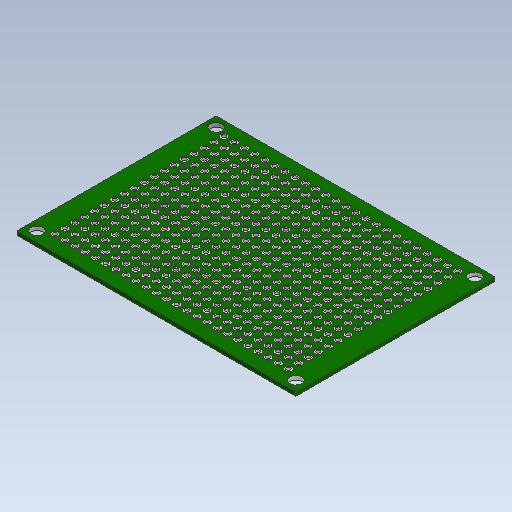
# Autodesk Inventor part: Lochrasterplatine50x70
Saved by Autodesk Inventor 2021 (Build 250183000, 183)
## iProperties
Created: 2020-12-16
Part Number: Lochrasterplatine50x70
Material: Generisch
Document SubType Name: Modeling
Designer: laure
Density: 1 g/cm^3
Appearance: Vorgabe
Author: laure
Autodesk Inventor part; units mm, degrees
(part 1 of 2)
ref_plane "YZ Plane" through (0, 0, 0) normal (1, 0, 0) x (0, 1, 0)
ref_plane "XZ Plane" through (0, 0, 0) normal (0, 1, 0) x (-1, 0, 0)
ref_plane "XY Plane" through (0, 0, 0) normal (0, 0, 1) x (1, 0, 0)
sketch "Skizze1" plane through (0, 0, 0) normal (0, 1, 0) x (-1, 0, 0)
  line L0 (-35, -25) -> (35, -25)
  line L1 (35, -25) -> (35, 25)
  line L2 (35, 25) -> (-35, 25)
  line L3 (-35, 25) -> (-35, -25)
  line L4 (0, -35) -> (0, 35) projected
  line L5 (49, 0) -> (-49, 0) projected
  point P0 (0, 0)
  dimension "d0" = 70
  dimension "d1" = 50
  constraints: 8 end point, 2 parallel, 1 horizontal, 1 perpendicular, 2 other
  measures "d0" distance of L1.end L2.end
  measures "d1" distance of L0.end L1.end
extrude "Extrusion1" add sketch "Skizze1" along normal mid plane 1
sketch "Skizze2" plane through (0, 0.5, 0) normal (0, 1, 0) x (1, 0, 0)
  circle A0 centre (-29.5, 21.5) radius 0.5
  line L0 (-35, 25) -> (-35, -25) projected
  line L1 (35, 25) -> (-35, 25) projected
  circle A1 centre (-26.95, 21.5) radius 0.5
  circle A2 centre (-24.4, 21.5) radius 0.5
  circle A3 centre (-21.85, 21.5) radius 0.5
  circle A4 centre (-19.3, 21.5) radius 0.5
  circle A5 centre (-16.75, 21.5) radius 0.5
  circle A6 centre (-14.2, 21.5) radius 0.5
  circle A7 centre (-11.65, 21.5) radius 0.5
  circle A8 centre (-9.1, 21.5) radius 0.5
  circle A9 centre (-6.55, 21.5) radius 0.5
  circle A10 centre (-4, 21.5) radius 0.5
  circle A11 centre (-1.45, 21.5) radius 0.5
  circle A12 centre (1.1, 21.5) radius 0.5
  circle A13 centre (3.65, 21.5) radius 0.5
  circle A14 centre (6.2, 21.5) radius 0.5
  circle A15 centre (8.75, 21.5) radius 0.5
  circle A16 centre (11.3, 21.5) radius 0.5
  circle A17 centre (13.85, 21.5) radius 0.5
  circle A18 centre (16.4, 21.5) radius 0.5
  circle A19 centre (18.95, 21.5) radius 0.5
  circle A20 centre (21.5, 21.5) radius 0.5
  circle A21 centre (24.05, 21.5) radius 0.5
  circle A22 centre (26.6, 21.5) radius 0.5
  circle A23 centre (29.15, 21.5) radius 0.5
  circle A24 centre (-29.5, 19) radius 0.5
  circle A25 centre (-26.95, 19) radius 0.5
  circle A26 centre (-24.4, 19) radius 0.5
  circle A27 centre (-21.85, 19) radius 0.5
  circle A28 centre (-19.3, 19) radius 0.5
  circle A29 centre (-16.75, 19) radius 0.5
  circle A30 centre (-14.2, 19) radius 0.5
  circle A31 centre (-11.65, 19) radius 0.5
  circle A32 centre (-9.1, 19) radius 0.5
  circle A33 centre (-6.55, 19) radius 0.5
  circle A34 centre (-4, 19) radius 0.5
  circle A35 centre (-1.45, 19) radius 0.5
  circle A36 centre (1.1, 19) radius 0.5
  circle A37 centre (3.65, 19) radius 0.5
  circle A38 centre (6.2, 19) radius 0.5
  circle A39 centre (8.75, 19) radius 0.5
  circle A40 centre (11.3, 19) radius 0.5
  circle A41 centre (13.85, 19) radius 0.5
  circle A42 centre (16.4, 19) radius 0.5
  circle A43 centre (18.95, 19) radius 0.5
  circle A44 centre (21.5, 19) radius 0.5
  circle A45 centre (24.05, 19) radius 0.5
  circle A46 centre (26.6, 19) radius 0.5
  circle A47 centre (29.15, 19) radius 0.5
  circle A48 centre (-29.5, 16.5) radius 0.5
  circle A49 centre (-26.95, 16.5) radius 0.5
  circle A50 centre (-24.4, 16.5) radius 0.5
  circle A51 centre (-21.85, 16.5) radius 0.5
  circle A52 centre (-19.3, 16.5) radius 0.5
  circle A53 centre (-16.75, 16.5) radius 0.5
  circle A54 centre (-14.2, 16.5) radius 0.5
  circle A55 centre (-11.65, 16.5) radius 0.5
  circle A56 centre (-9.1, 16.5) radius 0.5
  circle A57 centre (-6.55, 16.5) radius 0.5
  circle A58 centre (-4, 16.5) radius 0.5
  circle A59 centre (-1.45, 16.5) radius 0.5
  circle A60 centre (1.1, 16.5) radius 0.5
  circle A61 centre (3.65, 16.5) radius 0.5
  circle A62 centre (6.2, 16.5) radius 0.5
  circle A63 centre (8.75, 16.5) radius 0.5
  circle A64 centre (11.3, 16.5) radius 0.5
  circle A65 centre (13.85, 16.5) radius 0.5
  circle A66 centre (16.4, 16.5) radius 0.5
  circle A67 centre (18.95, 16.5) radius 0.5
  circle A68 centre (21.5, 16.5) radius 0.5
  circle A69 centre (24.05, 16.5) radius 0.5
  circle A70 centre (26.6, 16.5) radius 0.5
  circle A71 centre (29.15, 16.5) radius 0.5
  circle A72 centre (-29.5, 14) radius 0.5
  circle A73 centre (-26.95, 14) radius 0.5
  circle A74 centre (-24.4, 14) radius 0.5
  circle A75 centre (-21.85, 14) radius 0.5
  circle A76 centre (-19.3, 14) radius 0.5
  circle A77 centre (-16.75, 14) radius 0.5
  circle A78 centre (-14.2, 14) radius 0.5
  circle A79 centre (-11.65, 14) radius 0.5
  circle A80 centre (-9.1, 14) radius 0.5
  circle A81 centre (-6.55, 14) radius 0.5
  circle A82 centre (-4, 14) radius 0.5
  circle A83 centre (-1.45, 14) radius 0.5
  circle A84 centre (1.1, 14) radius 0.5
  circle A85 centre (3.65, 14) radius 0.5
  circle A86 centre (6.2, 14) radius 0.5
  circle A87 centre (8.75, 14) radius 0.5
  circle A88 centre (11.3, 14) radius 0.5
  circle A89 centre (13.85, 14) radius 0.5
  circle A90 centre (16.4, 14) radius 0.5
  circle A91 centre (18.95, 14) radius 0.5
  circle A92 centre (21.5, 14) radius 0.5
  circle A93 centre (24.05, 14) radius 0.5
  circle A94 centre (26.6, 14) radius 0.5
  circle A95 centre (29.15, 14) radius 0.5
  circle A96 centre (-29.5, 11.5) radius 0.5
  circle A97 centre (-26.95, 11.5) radius 0.5
  circle A98 centre (-24.4, 11.5) radius 0.5
  circle A99 centre (-21.85, 11.5) radius 0.5
  circle A100 centre (-19.3, 11.5) radius 0.5
  circle A101 centre (-16.75, 11.5) radius 0.5
  circle A102 centre (-14.2, 11.5) radius 0.5
  circle A103 centre (-11.65, 11.5) radius 0.5
  circle A104 centre (-9.1, 11.5) radius 0.5
  circle A105 centre (-6.55, 11.5) radius 0.5
  circle A106 centre (-4, 11.5) radius 0.5
  circle A107 centre (-1.45, 11.5) radius 0.5
  circle A108 centre (1.1, 11.5) radius 0.5
  circle A109 centre (3.65, 11.5) radius 0.5
  circle A110 centre (6.2, 11.5) radius 0.5
  circle A111 centre (8.75, 11.5) radius 0.5
  circle A112 centre (11.3, 11.5) radius 0.5
  circle A113 centre (13.85, 11.5) radius 0.5
  circle A114 centre (16.4, 11.5) radius 0.5
  circle A115 centre (18.95, 11.5) radius 0.5
  circle A116 centre (21.5, 11.5) radius 0.5
  circle A117 centre (24.05, 11.5) radius 0.5
  circle A118 centre (26.6, 11.5) radius 0.5
  circle A119 centre (29.15, 11.5) radius 0.5
  circle A120 centre (-29.5, 9) radius 0.5
  circle A121 centre (-26.95, 9) radius 0.5
  circle A122 centre (-24.4, 9) radius 0.5
  circle A123 centre (-21.85, 9) radius 0.5
  circle A124 centre (-19.3, 9) radius 0.5
  circle A125 centre (-16.75, 9) radius 0.5
  circle A126 centre (-14.2, 9) radius 0.5
  circle A127 centre (-11.65, 9) radius 0.5
  circle A128 centre (-9.1, 9) radius 0.5
  circle A129 centre (-6.55, 9) radius 0.5
  circle A130 centre (-4, 9) radius 0.5
  circle A131 centre (-1.45, 9) radius 0.5
  circle A132 centre (1.1, 9) radius 0.5
  circle A133 centre (3.65, 9) radius 0.5
  circle A134 centre (6.2, 9) radius 0.5
  circle A135 centre (8.75, 9) radius 0.5
  circle A136 centre (11.3, 9) radius 0.5
  circle A137 centre (13.85, 9) radius 0.5
  circle A138 centre (16.4, 9) radius 0.5
  circle A139 centre (18.95, 9) radius 0.5
  circle A140 centre (21.5, 9) radius 0.5
  circle A141 centre (24.05, 9) radius 0.5
  circle A142 centre (26.6, 9) radius 0.5
  circle A143 centre (29.15, 9) radius 0.5
  circle A144 centre (-29.5, 6.5) radius 0.5
  circle A145 centre (-26.95, 6.5) radius 0.5
  circle A146 centre (-24.4, 6.5) radius 0.5
  circle A147 centre (-21.85, 6.5) radius 0.5
  circle A148 centre (-19.3, 6.5) radius 0.5
  circle A149 centre (-16.75, 6.5) radius 0.5
  circle A150 centre (-14.2, 6.5) radius 0.5
  circle A151 centre (-11.65, 6.5) radius 0.5
  circle A152 centre (-9.1, 6.5) radius 0.5
  circle A153 centre (-6.55, 6.5) radius 0.5
  circle A154 centre (-4, 6.5) radius 0.5
  circle A155 centre (-1.45, 6.5) radius 0.5
  circle A156 centre (1.1, 6.5) radius 0.5
  circle A157 centre (3.65, 6.5) radius 0.5
  circle A158 centre (6.2, 6.5) radius 0.5
  circle A159 centre (8.75, 6.5) radius 0.5
  circle A160 centre (11.3, 6.5) radius 0.5
  circle A161 centre (13.85, 6.5) radius 0.5
  circle A162 centre (16.4, 6.5) radius 0.5
  circle A163 centre (18.95, 6.5) radius 0.5
  circle A164 centre (21.5, 6.5) radius 0.5
  circle A165 centre (24.05, 6.5) radius 0.5
  circle A166 centre (26.6, 6.5) radius 0.5
  circle A167 centre (29.15, 6.5) radius 0.5
  circle A168 centre (-29.5, 4) radius 0.5
  circle A169 centre (-26.95, 4) radius 0.5
  circle A170 centre (-24.4, 4) radius 0.5
  circle A171 centre (-21.85, 4) radius 0.5
  circle A172 centre (-19.3, 4) radius 0.5
  circle A173 centre (-16.75, 4) radius 0.5
  circle A174 centre (-14.2, 4) radius 0.5
  circle A175 centre (-11.65, 4) radius 0.5
  circle A176 centre (-9.1, 4) radius 0.5
  circle A177 centre (-6.55, 4) radius 0.5
  circle A178 centre (-4, 4) radius 0.5
  circle A179 centre (-1.45, 4) radius 0.5
  circle A180 centre (1.1, 4) radius 0.5
  circle A181 centre (3.65, 4) radius 0.5
  circle A182 centre (6.2, 4) radius 0.5
  circle A183 centre (8.75, 4) radius 0.5
  circle A184 centre (11.3, 4) radius 0.5
  circle A185 centre (13.85, 4) radius 0.5
  circle A186 centre (16.4, 4) radius 0.5
  circle A187 centre (18.95, 4) radius 0.5
  circle A188 centre (21.5, 4) radius 0.5
  circle A189 centre (24.05, 4) radius 0.5
  circle A190 centre (26.6, 4) radius 0.5
  circle A191 centre (29.15, 4) radius 0.5
  circle A192 centre (-29.5, 1.5) radius 0.5
  circle A193 centre (-26.95, 1.5) radius 0.5
  circle A194 centre (-24.4, 1.5) radius 0.5
  circle A195 centre (-21.85, 1.5) radius 0.5
  circle A196 centre (-19.3, 1.5) radius 0.5
  circle A197 centre (-16.75, 1.5) radius 0.5
  circle A198 centre (-14.2, 1.5) radius 0.5
  circle A199 centre (-11.65, 1.5) radius 0.5
  circle A200 centre (-9.1, 1.5) radius 0.5
  circle A201 centre (-6.55, 1.5) radius 0.5
  circle A202 centre (-4, 1.5) radius 0.5
  circle A203 centre (-1.45, 1.5) radius 0.5
  circle A204 centre (1.1, 1.5) radius 0.5
  circle A205 centre (3.65, 1.5) radius 0.5
  circle A206 centre (6.2, 1.5) radius 0.5
  circle A207 centre (8.75, 1.5) radius 0.5
  circle A208 centre (11.3, 1.5) radius 0.5
  circle A209 centre (13.85, 1.5) radius 0.5
  circle A210 centre (16.4, 1.5) radius 0.5
  circle A211 centre (18.95, 1.5) radius 0.5
  circle A212 centre (21.5, 1.5) radius 0.5
  circle A213 centre (24.05, 1.5) radius 0.5
  circle A214 centre (26.6, 1.5) radius 0.5
  circle A215 centre (29.15, 1.5) radius 0.5
  circle A216 centre (-29.5, -1) radius 0.5
  circle A217 centre (-26.95, -1) radius 0.5
  circle A218 centre (-24.4, -1) radius 0.5
  circle A219 centre (-21.85, -1) radius 0.5
  circle A220 centre (-19.3, -1) radius 0.5
  circle A221 centre (-16.75, -1) radius 0.5
  circle A222 centre (-14.2, -1) radius 0.5
  circle A223 centre (-11.65, -1) radius 0.5
  circle A224 centre (-9.1, -1) radius 0.5
  circle A225 centre (-6.55, -1) radius 0.5
  circle A226 centre (-4, -1) radius 0.5
  circle A227 centre (-1.45, -1) radius 0.5
  circle A228 centre (1.1, -1) radius 0.5
  circle A229 centre (3.65, -1) radius 0.5
  circle A230 centre (6.2, -1) radius 0.5
  circle A231 centre (8.75, -1) radius 0.5
  circle A232 centre (11.3, -1) radius 0.5
  circle A233 centre (13.85, -1) radius 0.5
  circle A234 centre (16.4, -1) radius 0.5
  circle A235 centre (18.95, -1) radius 0.5
  circle A236 centre (21.5, -1) radius 0.5
  circle A237 centre (24.05, -1) radius 0.5
  circle A238 centre (26.6, -1) radius 0.5
  circle A239 centre (29.15, -1) radius 0.5
  circle A240 centre (-29.5, -3.5) radius 0.5
  circle A241 centre (-26.95, -3.5) radius 0.5
  circle A242 centre (-24.4, -3.5) radius 0.5
  circle A243 centre (-21.85, -3.5) radius 0.5
  circle A244 centre (-19.3, -3.5) radius 0.5
  circle A245 centre (-16.75, -3.5) radius 0.5
  circle A246 centre (-14.2, -3.5) radius 0.5
  circle A247 centre (-11.65, -3.5) radius 0.5
  circle A248 centre (-9.1, -3.5) radius 0.5
  circle A249 centre (-6.55, -3.5) radius 0.5
  circle A250 centre (-4, -3.5) radius 0.5
  circle A251 centre (-1.45, -3.5) radius 0.5
  circle A252 centre (1.1, -3.5) radius 0.5
  circle A253 centre (3.65, -3.5) radius 0.5
  circle A254 centre (6.2, -3.5) radius 0.5
  circle A255 centre (8.75, -3.5) radius 0.5
  circle A256 centre (11.3, -3.5) radius 0.5
  circle A257 centre (13.85, -3.5) radius 0.5
  circle A258 centre (16.4, -3.5) radius 0.5
  circle A259 centre (18.95, -3.5) radius 0.5
  circle A260 centre (21.5, -3.5) radius 0.5
  circle A261 centre (24.05, -3.5) radius 0.5
  circle A262 centre (26.6, -3.5) radius 0.5
  circle A263 centre (29.15, -3.5) radius 0.5
  circle A264 centre (-29.5, -6) radius 0.5
  circle A265 centre (-26.95, -6) radius 0.5
  circle A266 centre (-24.4, -6) radius 0.5
  circle A267 centre (-21.85, -6) radius 0.5
  circle A268 centre (-19.3, -6) radius 0.5
  circle A269 centre (-16.75, -6) radius 0.5
  circle A270 centre (-14.2, -6) radius 0.5
  circle A271 centre (-11.65, -6) radius 0.5
  circle A272 centre (-9.1, -6) radius 0.5
  circle A273 centre (-6.55, -6) radius 0.5
  circle A274 centre (-4, -6) radius 0.5
  circle A275 centre (-1.45, -6) radius 0.5
  circle A276 centre (1.1, -6) radius 0.5
  circle A277 centre (3.65, -6) radius 0.5
  circle A278 centre (6.2, -6) radius 0.5
  circle A279 centre (8.75, -6) radius 0.5
  circle A280 centre (11.3, -6) radius 0.5
  circle A281 centre (13.85, -6) radius 0.5
  circle A282 centre (16.4, -6) radius 0.5
  circle A283 centre (18.95, -6) radius 0.5
  circle A284 centre (21.5, -6) radius 0.5
  circle A285 centre (24.05, -6) radius 0.5
  circle A286 centre (26.6, -6) radius 0.5
  circle A287 centre (29.15, -6) radius 0.5
  circle A288 centre (-29.5, -8.5) radius 0.5
  circle A289 centre (-26.95, -8.5) radius 0.5
  circle A290 centre (-24.4, -8.5) radius 0.5
  circle A291 centre (-21.85, -8.5) radius 0.5
  circle A292 centre (-19.3, -8.5) radius 0.5
  circle A293 centre (-16.75, -8.5) radius 0.5
  circle A294 centre (-14.2, -8.5) radius 0.5
  circle A295 centre (-11.65, -8.5) radius 0.5
  circle A296 centre (-9.1, -8.5) radius 0.5
  circle A297 centre (-6.55, -8.5) radius 0.5
  circle A298 centre (-4, -8.5) radius 0.5
  circle A299 centre (-1.45, -8.5) radius 0.5
  circle A300 centre (1.1, -8.5) radius 0.5
  circle A301 centre (3.65, -8.5) radius 0.5
  circle A302 centre (6.2, -8.5) radius 0.5
  circle A303 centre (8.75, -8.5) radius 0.5
  circle A304 centre (11.3, -8.5) radius 0.5
  circle A305 centre (13.85, -8.5) radius 0.5
  circle A306 centre (16.4, -8.5) radius 0.5
  circle A307 centre (18.95, -8.5) radius 0.5
  circle A308 centre (21.5, -8.5) radius 0.5
  circle A309 centre (24.05, -8.5) radius 0.5
  circle A310 centre (26.6, -8.5) radius 0.5
  circle A311 centre (29.15, -8.5) radius 0.5
  circle A312 centre (-29.5, -11) radius 0.5
  circle A313 centre (-26.95, -11) radius 0.5
  circle A314 centre (-24.4, -11) radius 0.5
  circle A315 centre (-21.85, -11) radius 0.5
  circle A316 centre (-19.3, -11) radius 0.5
  circle A317 centre (-16.75, -11) radius 0.5
  circle A318 centre (-14.2, -11) radius 0.5
  circle A319 centre (-11.65, -11) radius 0.5
  circle A320 centre (-9.1, -11) radius 0.5
  circle A321 centre (-6.55, -11) radius 0.5
  circle A322 centre (-4, -11) radius 0.5
  circle A323 centre (-1.45, -11) radius 0.5
  circle A324 centre (1.1, -11) radius 0.5
  circle A325 centre (3.65, -11) radius 0.5
  circle A326 centre (6.2, -11) radius 0.5
  circle A327 centre (8.75, -11) radius 0.5
  circle A328 centre (11.3, -11) radius 0.5
  circle A329 centre (13.85, -11) radius 0.5
  circle A330 centre (16.4, -11) radius 0.5
  circle A331 centre (18.95, -11) radius 0.5
  circle A332 centre (21.5, -11) radius 0.5
  circle A333 centre (24.05, -11) radius 0.5
  circle A334 centre (26.6, -11) radius 0.5
  circle A335 centre (29.15, -11) radius 0.5
  circle A336 centre (-29.5, -13.5) radius 0.5
  circle A337 centre (-26.95, -13.5) radius 0.5
  circle A338 centre (-24.4, -13.5) radius 0.5
  circle A339 centre (-21.85, -13.5) radius 0.5
  circle A340 centre (-19.3, -13.5) radius 0.5
  circle A341 centre (-16.75, -13.5) radius 0.5
  circle A342 centre (-14.2, -13.5) radius 0.5
  circle A343 centre (-11.65, -13.5) radius 0.5
  circle A344 centre (-9.1, -13.5) radius 0.5
  circle A345 centre (-6.55, -13.5) radius 0.5
  circle A346 centre (-4, -13.5) radius 0.5
  circle A347 centre (-1.45, -13.5) radius 0.5
  circle A348 centre (1.1, -13.5) radius 0.5
  circle A349 centre (3.65, -13.5) radius 0.5
  circle A350 centre (6.2, -13.5) radius 0.5
  circle A351 centre (8.75, -13.5) radius 0.5
  circle A352 centre (11.3, -13.5) radius 0.5
  circle A353 centre (13.85, -13.5) radius 0.5
  circle A354 centre (16.4, -13.5) radius 0.5
  circle A355 centre (18.95, -13.5) radius 0.5
  circle A356 centre (21.5, -13.5) radius 0.5
  circle A357 centre (24.05, -13.5) radius 0.5
  circle A358 centre (26.6, -13.5) radius 0.5
  circle A359 centre (29.15, -13.5) radius 0.5
  circle A360 centre (-29.5, -16) radius 0.5
  circle A361 centre (-26.95, -16) radius 0.5
  circle A362 centre (-24.4, -16) radius 0.5
  circle A363 centre (-21.85, -16) radius 0.5
  circle A364 centre (-19.3, -16) radius 0.5
  circle A365 centre (-16.75, -16) radius 0.5
  circle A366 centre (-14.2, -16) radius 0.5
  circle A367 centre (-11.65, -16) radius 0.5
  circle A368 centre (-9.1, -16) radius 0.5
  circle A369 centre (-6.55, -16) radius 0.5
  circle A370 centre (-4, -16) radius 0.5
  circle A371 centre (-1.45, -16) radius 0.5
  circle A372 centre (1.1, -16) radius 0.5
  circle A373 centre (3.65, -16) radius 0.5
  circle A374 centre (6.2, -16) radius 0.5
  circle A375 centre (8.75, -16) radius 0.5
  circle A376 centre (11.3, -16) radius 0.5
  circle A377 centre (13.85, -16) radius 0.5
  circle A378 centre (16.4, -16) radius 0.5
  circle A379 centre (18.95, -16) radius 0.5
  circle A380 centre (21.5, -16) radius 0.5
  circle A381 centre (24.05, -16) radius 0.5
  circle A382 centre (26.6, -16) radius 0.5
  circle A383 centre (29.15, -16) radius 0.5
  circle A384 centre (-29.5, -18.5) radius 0.5
  circle A385 centre (-26.95, -18.5) radius 0.5
  circle A386 centre (-24.4, -18.5) radius 0.5
  circle A387 centre (-21.85, -18.5) radius 0.5
  circle A388 centre (-19.3, -18.5) radius 0.5
  circle A389 centre (-16.75, -18.5) radius 0.5
  circle A390 centre (-14.2, -18.5) radius 0.5
  circle A391 centre (-11.65, -18.5) radius 0.5
  circle A392 centre (-9.1, -18.5) radius 0.5
  circle A393 centre (-6.55, -18.5) radius 0.5
  circle A394 centre (-4, -18.5) radius 0.5
  circle A395 centre (-1.45, -18.5) radius 0.5
  circle A396 centre (1.1, -18.5) radius 0.5
  circle A397 centre (3.65, -18.5) radius 0.5
  circle A398 centre (6.2, -18.5) radius 0.5
  circle A399 centre (8.75, -18.5) radius 0.5
  circle A400 centre (11.3, -18.5) radius 0.5
  circle A401 centre (13.85, -18.5) radius 0.5
  circle A402 centre (16.4, -18.5) radius 0.5
  circle A403 centre (18.95, -18.5) radius 0.5
  circle A404 centre (21.5, -18.5) radius 0.5
  circle A405 centre (24.05, -18.5) radius 0.5
  circle A406 centre (26.6, -18.5) radius 0.5
  circle A407 centre (29.15, -18.5) radius 0.5
  circle A408 centre (-29.5, -21) radius 0.5
  circle A409 centre (-26.95, -21) radius 0.5
  circle A410 centre (-24.4, -21) radius 0.5
  circle A411 centre (-21.85, -21) radius 0.5
  circle A412 centre (-19.3, -21) radius 0.5
  circle A413 centre (-16.75, -21) radius 0.5
  circle A414 centre (-14.2, -21) radius 0.5
  circle A415 centre (-11.65, -21) radius 0.5
  circle A416 centre (-9.1, -21) radius 0.5
  circle A417 centre (-6.55, -21) radius 0.5
  circle A418 centre (-4, -21) radius 0.5
  circle A419 centre (-1.45, -21) radius 0.5
  circle A420 centre (1.1, -21) radius 0.5
  circle A421 centre (3.65, -21) radius 0.5
  circle A422 centre (6.2, -21) radius 0.5
  circle A423 centre (8.75, -21) radius 0.5
  circle A424 centre (11.3, -21) radius 0.5
  circle A425 centre (13.85, -21) radius 0.5
  circle A426 centre (16.4, -21) radius 0.5
  circle A427 centre (18.95, -21) radius 0.5
  circle A428 centre (21.5, -21) radius 0.5
  circle A429 centre (24.05, -21) radius 0.5
  circle A430 centre (26.6, -21) radius 0.5
  circle A431 centre (29.15, -21) radius 0.5
  dimension "d5" = 5.5
  dimension "d24" = 2.55
  dimension "d27" = 2.5
  constraints: 432 centre point, 1 horizontal, 1 vertical, 862 other
  measures "d5" distance from line of L0 A0.centre
  measures "d24" distance of A0.centre A1.centre
  measures "d27" distance of A0.centre A24.centre
sketch "Skizze3" plane through (0, 0.5, 0) normal (0, 1, 0) x (1, 0, 0)
  circle A0 centre (-32.5, 22.5) radius 1.5
  line L0 (-35, 25) -> (-35, -25) projected
  line L1 (35, 25) -> (-35, 25) projected
  line L2 (-35, -25) -> (-35, 25) projected
  line L3 (-35, 0) -> (35, 0)
  line L4 (35, -25) -> (35, 25) projected
  line L5 (0, 25) -> (0, -25.4549)
  line L6 (35, -25) -> (-35, -25) projected
  circle A1 centre (-32.5, -22.5) radius 1.5
  circle A2 centre (32.5, 22.5) radius 1.5
  circle A3 centre (32.5, -22.5) radius 1.5
  point P0 (0, 0)
  dimension "d17" = 3
  dimension "d18" = 2.5
  dimension "d19" = 2.5
  constraints: 4 centre point, 4 end point, 3 midpoint, 3 symmetric about line, 1 perpendicular, 3 other
  measures "d17" diameter of A0
  measures "d18" distance from line of L0 A0.centre
  measures "d19" distance from line of L1 A0.centre
extrude "Extrusion3" cut sketch "Skizze3" against normal blind 1 contours A0 | A1 | A2 | A3
extrude "Extrusion4" cut sketch "Skizze2" against normal blind 1
sketch "Skizze4" plane through (0, 0.5, 0) normal (0, 1, 0) x (1, 0, 0)
  circle A0 centre (-29.5, 21.5) radius 0.5 projected
  circle A1 centre (-29.5, 21.5) radius 0.875
  line L0 (-35, -25) -> (-35, 25) projected
  line L1 (-35, 25) -> (35, 25) projected
  line L2 (-35, 25) -> (35, 25)
  line L3 (35, -25) -> (-35, -25) projected
  line L4 (-35, 25) -> (-35, -25)
  circle A2 centre (-26.95, 21.5) radius 0.875
  circle A3 centre (-24.4, 21.5) radius 0.875
  circle A4 centre (-21.85, 21.5) radius 0.875
  circle A5 centre (-19.3, 21.5) radius 0.875
  circle A6 centre (-16.75, 21.5) radius 0.875
  circle A7 centre (-14.2, 21.5) radius 0.875
  circle A8 centre (-11.65, 21.5) radius 0.875
  circle A9 centre (-9.1, 21.5) radius 0.875
  circle A10 centre (-6.55, 21.5) radius 0.875
  circle A11 centre (-4, 21.5) radius 0.875
  circle A12 centre (-1.45, 21.5) radius 0.875
  circle A13 centre (1.1, 21.5) radius 0.875
  circle A14 centre (3.65, 21.5) radius 0.875
  circle A15 centre (6.2, 21.5) radius 0.875
  circle A16 centre (8.75, 21.5) radius 0.875
  circle A17 centre (11.3, 21.5) radius 0.875
  circle A18 centre (13.85, 21.5) radius 0.875
  circle A19 centre (16.4, 21.5) radius 0.875
  circle A20 centre (18.95, 21.5) radius 0.875
  circle A21 centre (21.5, 21.5) radius 0.875
  circle A22 centre (24.05, 21.5) radius 0.875
  circle A23 centre (26.6, 21.5) radius 0.875
  circle A24 centre (29.15, 21.5) radius 0.875
  circle A25 centre (-29.5, 19) radius 0.875
  circle A26 centre (-26.95, 19) radius 0.875
  circle A27 centre (-24.4, 19) radius 0.875
  circle A28 centre (-21.85, 19) radius 0.875
  circle A29 centre (-19.3, 19) radius 0.875
  circle A30 centre (-16.75, 19) radius 0.875
  circle A31 centre (-14.2, 19) radius 0.875
  circle A32 centre (-11.65, 19) radius 0.875
  circle A33 centre (-9.1, 19) radius 0.875
  circle A34 centre (-6.55, 19) radius 0.875
  circle A35 centre (-4, 19) radius 0.875
  circle A36 centre (-1.45, 19) radius 0.875
  circle A37 centre (1.1, 19) radius 0.875
  circle A38 centre (3.65, 19) radius 0.875
  circle A39 centre (6.2, 19) radius 0.875
  circle A40 centre (8.75, 19) radius 0.875
  circle A41 centre (11.3, 19) radius 0.875
  circle A42 centre (13.85, 19) radius 0.875
  circle A43 centre (16.4, 19) radius 0.875
  circle A44 centre (18.95, 19) radius 0.875
  circle A45 centre (21.5, 19) radius 0.875
  circle A46 centre (24.05, 19) radius 0.875
  circle A47 centre (26.6, 19) radius 0.875
  circle A48 centre (29.15, 19) radius 0.875
  circle A49 centre (-29.5, 16.5) radius 0.875
  circle A50 centre (-26.95, 16.5) radius 0.875
  circle A51 centre (-24.4, 16.5) radius 0.875
  circle A52 centre (-21.85, 16.5) radius 0.875
  circle A53 centre (-19.3, 16.5) radius 0.875
  circle A54 centre (-16.75, 16.5) radius 0.875
  circle A55 centre (-14.2, 16.5) radius 0.875
  circle A56 centre (-11.65, 16.5) radius 0.875
  circle A57 centre (-9.1, 16.5) radius 0.875
  circle A58 centre (-6.55, 16.5) radius 0.875
  circle A59 centre (-4, 16.5) radius 0.875
  circle A60 centre (-1.45, 16.5) radius 0.875
  circle A61 centre (1.1, 16.5) radius 0.875
  circle A62 centre (3.65, 16.5) radius 0.875
  circle A63 centre (6.2, 16.5) radius 0.875
  circle A64 centre (8.75, 16.5) radius 0.875
  circle A65 centre (11.3, 16.5) radius 0.875
  circle A66 centre (13.85, 16.5) radius 0.875
  circle A67 centre (16.4, 16.5) radius 0.875
  circle A68 centre (18.95, 16.5) radius 0.875
  circle A69 centre (21.5, 16.5) radius 0.875
  circle A70 centre (24.05, 16.5) radius 0.875
  circle A71 centre (26.6, 16.5) radius 0.875
  circle A72 centre (29.15, 16.5) radius 0.875
  circle A73 centre (-29.5, 14) radius 0.875
  circle A74 centre (-26.95, 14) radius 0.875
  circle A75 centre (-24.4, 14) radius 0.875
  circle A76 centre (-21.85, 14) radius 0.875
  circle A77 centre (-19.3, 14) radius 0.875
  circle A78 centre (-16.75, 14) radius 0.875
  circle A79 centre (-14.2, 14) radius 0.875
  circle A80 centre (-11.65, 14) radius 0.875
  circle A81 centre (-9.1, 14) radius 0.875
  circle A82 centre (-6.55, 14) radius 0.875
  circle A83 centre (-4, 14) radius 0.875
  circle A84 centre (-1.45, 14) radius 0.875
  circle A85 centre (1.1, 14) radius 0.875
  circle A86 centre (3.65, 14) radius 0.875
  circle A87 centre (6.2, 14) radius 0.875
  circle A88 centre (8.75, 14) radius 0.875
  circle A89 centre (11.3, 14) radius 0.875
  circle A90 centre (13.85, 14) radius 0.875
  circle A91 centre (16.4, 14) radius 0.875
  circle A92 centre (18.95, 14) radius 0.875
  circle A93 centre (21.5, 14) radius 0.875
  circle A94 centre (24.05, 14) radius 0.875
  circle A95 centre (26.6, 14) radius 0.875
  circle A96 centre (29.15, 14) radius 0.875
  circle A97 centre (-29.5, 11.5) radius 0.875
  circle A98 centre (-26.95, 11.5) radius 0.875
  circle A99 centre (-24.4, 11.5) radius 0.875
  circle A100 centre (-21.85, 11.5) radius 0.875
  circle A101 centre (-19.3, 11.5) radius 0.875
  circle A102 centre (-16.75, 11.5) radius 0.875
  circle A103 centre (-14.2, 11.5) radius 0.875
  circle A104 centre (-11.65, 11.5) radius 0.875
  circle A105 centre (-9.1, 11.5) radius 0.875
  circle A106 centre (-6.55, 11.5) radius 0.875
  circle A107 centre (-4, 11.5) radius 0.875
  circle A108 centre (-1.45, 11.5) radius 0.875
  circle A109 centre (1.1, 11.5) radius 0.875
  circle A110 centre (3.65, 11.5) radius 0.875
  circle A111 centre (6.2, 11.5) radius 0.875
  circle A112 centre (8.75, 11.5) radius 0.875
  circle A113 centre (11.3, 11.5) radius 0.875
  circle A114 centre (13.85, 11.5) radius 0.875
  circle A115 centre (16.4, 11.5) radius 0.875
  circle A116 centre (18.95, 11.5) radius 0.875
  circle A117 centre (21.5, 11.5) radius 0.875
  circle A118 centre (24.05, 11.5) radius 0.875
  circle A119 centre (26.6, 11.5) radius 0.875
  circle A120 centre (29.15, 11.5) radius 0.875
  circle A121 centre (-29.5, 9) radius 0.875
  circle A122 centre (-26.95, 9) radius 0.875
  circle A123 centre (-24.4, 9) radius 0.875
  circle A124 centre (-21.85, 9) radius 0.875
  circle A125 centre (-19.3, 9) radius 0.875
  circle A126 centre (-16.75, 9) radius 0.875
  circle A127 centre (-14.2, 9) radius 0.875
  circle A128 centre (-11.65, 9) radius 0.875
  circle A129 centre (-9.1, 9) radius 0.875
  circle A130 centre (-6.55, 9) radius 0.875
  circle A131 centre (-4, 9) radius 0.875
  circle A132 centre (-1.45, 9) radius 0.875
  circle A133 centre (1.1, 9) radius 0.875
  circle A134 centre (3.65, 9) radius 0.875
  circle A135 centre (6.2, 9) radius 0.875
  circle A136 centre (8.75, 9) radius 0.875
  circle A137 centre (11.3, 9) radius 0.875
  circle A138 centre (13.85, 9) radius 0.875
  circle A139 centre (16.4, 9) radius 0.875
  circle A140 centre (18.95, 9) radius 0.875
  circle A141 centre (21.5, 9) radius 0.875
  circle A142 centre (24.05, 9) radius 0.875
  circle A143 centre (26.6, 9) radius 0.875
  circle A144 centre (29.15, 9) radius 0.875
  circle A145 centre (-29.5, 6.5) radius 0.875
  circle A146 centre (-26.95, 6.5) radius 0.875
  circle A147 centre (-24.4, 6.5) radius 0.875
  circle A148 centre (-21.85, 6.5) radius 0.875
  circle A149 centre (-19.3, 6.5) radius 0.875
  circle A150 centre (-16.75, 6.5) radius 0.875
  circle A151 centre (-14.2, 6.5) radius 0.875
  circle A152 centre (-11.65, 6.5) radius 0.875
  circle A153 centre (-9.1, 6.5) radius 0.875
  circle A154 centre (-6.55, 6.5) radius 0.875
  circle A155 centre (-4, 6.5) radius 0.875
  circle A156 centre (-1.45, 6.5) radius 0.875
  circle A157 centre (1.1, 6.5) radius 0.875
  circle A158 centre (3.65, 6.5) radius 0.875
  circle A159 centre (6.2, 6.5) radius 0.875
  circle A160 centre (8.75, 6.5) radius 0.875
  circle A161 centre (11.3, 6.5) radius 0.875
  circle A162 centre (13.85, 6.5) radius 0.875
  circle A163 centre (16.4, 6.5) radius 0.875
  circle A164 centre (18.95, 6.5) radius 0.875
  circle A165 centre (21.5, 6.5) radius 0.875
  circle A166 centre (24.05, 6.5) radius 0.875
  circle A167 centre (26.6, 6.5) radius 0.875
  circle A168 centre (29.15, 6.5) radius 0.875
  circle A169 centre (-29.5, 4) radius 0.875
  circle A170 centre (-26.95, 4) radius 0.875
  circle A171 centre (-24.4, 4) radius 0.875
  circle A172 centre (-21.85, 4) radius 0.875
  circle A173 centre (-19.3, 4) radius 0.875
  circle A174 centre (-16.75, 4) radius 0.875
  circle A175 centre (-14.2, 4) radius 0.875
  circle A176 centre (-11.65, 4) radius 0.875
  circle A177 centre (-9.1, 4) radius 0.875
  circle A178 centre (-6.55, 4) radius 0.875
  circle A179 centre (-4, 4) radius 0.875
  circle A180 centre (-1.45, 4) radius 0.875
  circle A181 centre (1.1, 4) radius 0.875
  circle A182 centre (3.65, 4) radius 0.875
  circle A183 centre (6.2, 4) radius 0.875
  circle A184 centre (8.75, 4) radius 0.875
  circle A185 centre (11.3, 4) radius 0.875
  circle A186 centre (13.85, 4) radius 0.875
  circle A187 centre (16.4, 4) radius 0.875
  circle A188 centre (18.95, 4) radius 0.875
  circle A189 centre (21.5, 4) radius 0.875
  circle A190 centre (24.05, 4) radius 0.875
  circle A191 centre (26.6, 4) radius 0.875
  circle A192 centre (29.15, 4) radius 0.875
  circle A193 centre (-29.5, 1.5) radius 0.875
  circle A194 centre (-26.95, 1.5) radius 0.875
  circle A195 centre (-24.4, 1.5) radius 0.875
  circle A196 centre (-21.85, 1.5) radius 0.875
  circle A197 centre (-19.3, 1.5) radius 0.875
  circle A198 centre (-16.75, 1.5) radius 0.875
  circle A199 centre (-14.2, 1.5) radius 0.875
  circle A200 centre (-11.65, 1.5) radius 0.875
  circle A201 centre (-9.1, 1.5) radius 0.875
  circle A202 centre (-6.55, 1.5) radius 0.875
  circle A203 centre (-4, 1.5) radius 0.875
  circle A204 centre (-1.45, 1.5) radius 0.875
  circle A205 centre (1.1, 1.5) radius 0.875
  circle A206 centre (3.65, 1.5) radius 0.875
  circle A207 centre (6.2, 1.5) radius 0.875
  circle A208 centre (8.75, 1.5) radius 0.875
  circle A209 centre (11.3, 1.5) radius 0.875
  circle A210 centre (13.85, 1.5) radius 0.875
  circle A211 centre (16.4, 1.5) radius 0.875
  circle A212 centre (18.95, 1.5) radius 0.875
  circle A213 centre (21.5, 1.5) radius 0.875
  circle A214 centre (24.05, 1.5) radius 0.875
  circle A215 centre (26.6, 1.5) radius 0.875
  circle A216 centre (29.15, 1.5) radius 0.875
  circle A217 centre (-29.5, -1) radius 0.875
  circle A218 centre (-26.95, -1) radius 0.875
  circle A219 centre (-24.4, -1) radius 0.875
  circle A220 centre (-21.85, -1) radius 0.875
  circle A221 centre (-19.3, -1) radius 0.875
  circle A222 centre (-16.75, -1) radius 0.875
  circle A223 centre (-14.2, -1) radius 0.875
  circle A224 centre (-11.65, -1) radius 0.875
  circle A225 centre (-9.1, -1) radius 0.875
  circle A226 centre (-6.55, -1) radius 0.875
  circle A227 centre (-4, -1) radius 0.875
  circle A228 centre (-1.45, -1) radius 0.875
  circle A229 centre (1.1, -1) radius 0.875
  circle A230 centre (3.65, -1) radius 0.875
  circle A231 centre (6.2, -1) radius 0.875
  circle A232 centre (8.75, -1) radius 0.875
  circle A233 centre (11.3, -1) radius 0.875
  circle A234 centre (13.85, -1) radius 0.875
  circle A235 centre (16.4, -1) radius 0.875
  circle A236 centre (18.95, -1) radius 0.875
  circle A237 centre (21.5, -1) radius 0.875
  circle A238 centre (24.05, -1) radius 0.875
  circle A239 centre (26.6, -1) radius 0.875
  circle A240 centre (29.15, -1) radius 0.875
  circle A241 centre (-29.5, -3.5) radius 0.875
  circle A242 centre (-26.95, -3.5) radius 0.875
  circle A243 centre (-24.4, -3.5) radius 0.875
  circle A244 centre (-21.85, -3.5) radius 0.875
  circle A245 centre (-19.3, -3.5) radius 0.875
  circle A246 centre (-16.75, -3.5) radius 0.875
  circle A247 centre (-14.2, -3.5) radius 0.875
  circle A248 centre (-11.65, -3.5) radius 0.875
  circle A249 centre (-9.1, -3.5) radius 0.875
  circle A250 centre (-6.55, -3.5) radius 0.875
  circle A251 centre (-4, -3.5) radius 0.875
  circle A252 centre (-1.45, -3.5) radius 0.875
  circle A253 centre (1.1, -3.5) radius 0.875
  circle A254 centre (3.65, -3.5) radius 0.875
  circle A255 centre (6.2, -3.5) radius 0.875
  circle A256 centre (8.75, -3.5) radius 0.875
  circle A257 centre (11.3, -3.5) radius 0.875
  circle A258 centre (13.85, -3.5) radius 0.875
  circle A259 centre (16.4, -3.5) radius 0.875
  circle A260 centre (18.95, -3.5) radius 0.875
  circle A261 centre (21.5, -3.5) radius 0.875
  circle A262 centre (24.05, -3.5) radius 0.875
  circle A263 centre (26.6, -3.5) radius 0.875
  circle A264 centre (29.15, -3.5) radius 0.875
  circle A265 centre (-29.5, -6) radius 0.875
  circle A266 centre (-26.95, -6) radius 0.875
  circle A267 centre (-24.4, -6) radius 0.875
  circle A268 centre (-21.85, -6) radius 0.875
  circle A269 centre (-19.3, -6) radius 0.875
  circle A270 centre (-16.75, -6) radius 0.875
  circle A271 centre (-14.2, -6) radius 0.875
  circle A272 centre (-11.65, -6) radius 0.875
  circle A273 centre (-9.1, -6) radius 0.875
  circle A274 centre (-6.55, -6) radius 0.875
  circle A275 centre (-4, -6) radius 0.875
  circle A276 centre (-1.45, -6) radius 0.875
  circle A277 centre (1.1, -6) radius 0.875
  circle A278 centre (3.65, -6) radius 0.875
  circle A279 centre (6.2, -6) radius 0.875
  circle A280 centre (8.75, -6) radius 0.875
  circle A281 centre (11.3, -6) radius 0.875
  circle A282 centre (13.85, -6) radius 0.875
  circle A283 centre (16.4, -6) radius 0.875
  circle A284 centre (18.95, -6) radius 0.875
  circle A285 centre (21.5, -6) radius 0.875
  circle A286 centre (24.05, -6) radius 0.875
  circle A287 centre (26.6, -6) radius 0.875
  circle A288 centre (29.15, -6) radius 0.875
  circle A289 centre (-29.5, -8.5) radius 0.875
  circle A290 centre (-26.95, -8.5) radius 0.875
  circle A291 centre (-24.4, -8.5) radius 0.875
  circle A292 centre (-21.85, -8.5) radius 0.875
  circle A293 centre (-19.3, -8.5) radius 0.875
  circle A294 centre (-16.75, -8.5) radius 0.875
  circle A295 centre (-14.2, -8.5) radius 0.875
  circle A296 centre (-11.65, -8.5) radius 0.875
  circle A297 centre (-9.1, -8.5) radius 0.875
  circle A298 centre (-6.55, -8.5) radius 0.875
  circle A299 centre (-4, -8.5) radius 0.875
  circle A300 centre (-1.45, -8.5) radius 0.875
  circle A301 centre (1.1, -8.5) radius 0.875
  circle A302 centre (3.65, -8.5) radius 0.875
  circle A303 centre (6.2, -8.5) radius 0.875
  circle A304 centre (8.75, -8.5) radius 0.875
  circle A305 centre (11.3, -8.5) radius 0.875
  circle A306 centre (13.85, -8.5) radius 0.875
  circle A307 centre (16.4, -8.5) radius 0.875
  circle A308 centre (18.95, -8.5) radius 0.875
  circle A309 centre (21.5, -8.5) radius 0.875
  circle A310 centre (24.05, -8.5) radius 0.875
  circle A311 centre (26.6, -8.5) radius 0.875
  circle A312 centre (29.15, -8.5) radius 0.875
  circle A313 centre (-29.5, -11) radius 0.875
  circle A314 centre (-26.95, -11) radius 0.875
  circle A315 centre (-24.4, -11) radius 0.875
  circle A316 centre (-21.85, -11) radius 0.875
  circle A317 centre (-19.3, -11) radius 0.875
  circle A318 centre (-16.75, -11) radius 0.875
  circle A319 centre (-14.2, -11) radius 0.875
  circle A320 centre (-11.65, -11) radius 0.875
  circle A321 centre (-9.1, -11) radius 0.875
  circle A322 centre (-6.55, -11) radius 0.875
  circle A323 centre (-4, -11) radius 0.875
  circle A324 centre (-1.45, -11) radius 0.875
  circle A325 centre (1.1, -11) radius 0.875
  circle A326 centre (3.65, -11) radius 0.875
  circle A327 centre (6.2, -11) radius 0.875
  circle A328 centre (8.75, -11) radius 0.875
  circle A329 centre (11.3, -11) radius 0.875
  circle A330 centre (13.85, -11) radius 0.875
  circle A331 centre (16.4, -11) radius 0.875
  circle A332 centre (18.95, -11) radius 0.875
  circle A333 centre (21.5, -11) radius 0.875
  circle A334 centre (24.05, -11) radius 0.875
  circle A335 centre (26.6, -11) radius 0.875
  circle A336 centre (29.15, -11) radius 0.875
  circle A337 centre (-29.5, -13.5) radius 0.875
  circle A338 centre (-26.95, -13.5) radius 0.875
  circle A339 centre (-24.4, -13.5) radius 0.875
  circle A340 centre (-21.85, -13.5) radius 0.875
  circle A341 centre (-19.3, -13.5) radius 0.875
  circle A342 centre (-16.75, -13.5) radius 0.875
  circle A343 centre (-14.2, -13.5) radius 0.875
  circle A344 centre (-11.65, -13.5) radius 0.875
  circle A345 centre (-9.1, -13.5) radius 0.875
  circle A346 centre (-6.55, -13.5) radius 0.875
  circle A347 centre (-4, -13.5) radius 0.875
  circle A348 centre (-1.45, -13.5) radius 0.875
  circle A349 centre (1.1, -13.5) radius 0.875
  circle A350 centre (3.65, -13.5) radius 0.875
  circle A351 centre (6.2, -13.5) radius 0.875
  circle A352 centre (8.75, -13.5) radius 0.875
  circle A353 centre (11.3, -13.5) radius 0.875
  circle A354 centre (13.85, -13.5) radius 0.875
  circle A355 centre (16.4, -13.5) radius 0.875
  circle A356 centre (18.95, -13.5) radius 0.875
  circle A357 centre (21.5, -13.5) radius 0.875
  circle A358 centre (24.05, -13.5) radius 0.875
  circle A359 centre (26.6, -13.5) radius 0.875
  circle A360 centre (29.15, -13.5) radius 0.875
  circle A361 centre (-29.5, -16) radius 0.875
  circle A362 centre (-26.95, -16) radius 0.875
  circle A363 centre (-24.4, -16) radius 0.875
  circle A364 centre (-21.85, -16) radius 0.875
  circle A365 centre (-19.3, -16) radius 0.875
  circle A366 centre (-16.75, -16) radius 0.875
  circle A367 centre (-14.2, -16) radius 0.875
  circle A368 centre (-11.65, -16) radius 0.875
  circle A369 centre (-9.1, -16) radius 0.875
  circle A370 centre (-6.55, -16) radius 0.875
  circle A371 centre (-4, -16) radius 0.875
  circle A372 centre (-1.45, -16) radius 0.875
  circle A373 centre (1.1, -16) radius 0.875
  circle A374 centre (3.65, -16) radius 0.875
  circle A375 centre (6.2, -16) radius 0.875
  circle A376 centre (8.75, -16) radius 0.875
  circle A377 centre (11.3, -16) radius 0.875
  circle A378 centre (13.85, -16) radius 0.875
  circle A379 centre (16.4, -16) radius 0.875
  circle A380 centre (18.95, -16) radius 0.875
  circle A381 centre (21.5, -16) radius 0.875
  circle A382 centre (24.05, -16) radius 0.875
  circle A383 centre (26.6, -16) radius 0.875
  circle A384 centre (29.15, -16) radius 0.875
  circle A385 centre (-29.5, -18.5) radius 0.875
  circle A386 centre (-26.95, -18.5) radius 0.875
  circle A387 centre (-24.4, -18.5) radius 0.875
  circle A388 centre (-21.85, -18.5) radius 0.875
  circle A389 centre (-19.3, -18.5) radius 0.875
  circle A390 centre (-16.75, -18.5) radius 0.875
  circle A391 centre (-14.2, -18.5) radius 0.875
  circle A392 centre (-11.65, -18.5) radius 0.875
  circle A393 centre (-9.1, -18.5) radius 0.875
  circle A394 centre (-6.55, -18.5) radius 0.875
  circle A395 centre (-4, -18.5) radius 0.875
  circle A396 centre (-1.45, -18.5) radius 0.875
  circle A397 centre (1.1, -18.5) radius 0.875
  circle A398 centre (3.65, -18.5) radius 0.875
  circle A399 centre (6.2, -18.5) radius 0.875
  circle A400 centre (8.75, -18.5) radius 0.875
  circle A401 centre (11.3, -18.5) radius 0.875
  circle A402 centre (13.85, -18.5) radius 0.875
  circle A403 centre (16.4, -18.5) radius 0.875
  circle A404 centre (18.95, -18.5) radius 0.875
  circle A405 centre (21.5, -18.5) radius 0.875
  circle A406 centre (24.05, -18.5) radius 0.875
  circle A407 centre (26.6, -18.5) radius 0.875
  circle A408 centre (29.15, -18.5) radius 0.875
  circle A409 centre (-29.5, -21) radius 0.875
  circle A410 centre (-26.95, -21) radius 0.875
  circle A411 centre (-24.4, -21) radius 0.875
  circle A412 centre (-21.85, -21) radius 0.875
  circle A413 centre (-19.3, -21) radius 0.875
  circle A414 centre (-16.75, -21) radius 0.875
  circle A415 centre (-14.2, -21) radius 0.875
  circle A416 centre (-11.65, -21) radius 0.875
  circle A417 centre (-9.1, -21) radius 0.875
  circle A418 centre (-6.55, -21) radius 0.875
  circle A419 centre (-4, -21) radius 0.875
  circle A420 centre (-1.45, -21) radius 0.875
  circle A421 centre (1.1, -21) radius 0.875
  circle A422 centre (3.65, -21) radius 0.875
  circle A423 centre (6.2, -21) radius 0.875
  circle A424 centre (8.75, -21) radius 0.875
  circle A425 centre (11.3, -21) radius 0.875
  circle A426 centre (13.85, -21) radius 0.875
  circle A427 centre (16.4, -21) radius 0.875
  circle A428 centre (18.95, -21) radius 0.875
  circle A429 centre (21.5, -21) radius 0.875
  circle A430 centre (24.05, -21) radius 0.875
  circle A431 centre (26.6, -21) radius 0.875
  circle A432 centre (29.15, -21) radius 0.875
  circle A433 centre (-29.5, 21.5) radius 0.5
  circle A434 centre (-26.95, 21.5) radius 0.5
  circle A435 centre (-24.4, 21.5) radius 0.5
  circle A436 centre (-21.85, 21.5) radius 0.5
  circle A437 centre (-19.3, 21.5) radius 0.5
  circle A438 centre (-16.75, 21.5) radius 0.5
  circle A439 centre (-14.2, 21.5) radius 0.5
  circle A440 centre (-11.65, 21.5) radius 0.5
  circle A441 centre (-9.1, 21.5) radius 0.5
  circle A442 centre (-6.55, 21.5) radius 0.5
  circle A443 centre (-4, 21.5) radius 0.5
  circle A444 centre (-1.45, 21.5) radius 0.5
  circle A445 centre (1.1, 21.5) radius 0.5
  circle A446 centre (3.65, 21.5) radius 0.5
  circle A447 centre (6.2, 21.5) radius 0.5
  circle A448 centre (8.75, 21.5) radius 0.5
  circle A449 centre (11.3, 21.5) radius 0.5
  circle A450 centre (13.85, 21.5) radius 0.5
  circle A451 centre (16.4, 21.5) radius 0.5
  circle A452 centre (18.95, 21.5) radius 0.5
  circle A453 centre (21.5, 21.5) radius 0.5
  circle A454 centre (24.05, 21.5) radius 0.5
  circle A455 centre (26.6, 21.5) radius 0.5
  circle A456 centre (29.15, 21.5) radius 0.5
  circle A457 centre (-29.5, 19) radius 0.5
  circle A458 centre (-26.95, 19) radius 0.5
  circle A459 centre (-24.4, 19) radius 0.5
  circle A460 centre (-21.85, 19) radius 0.5
  circle A461 centre (-19.3, 19) radius 0.5
  circle A462 centre (-16.75, 19) radius 0.5
  circle A463 centre (-14.2, 19) radius 0.5
  circle A464 centre (-11.65, 19) radius 0.5
  circle A465 centre (-9.1, 19) radius 0.5
  circle A466 centre (-6.55, 19) radius 0.5
  circle A467 centre (-4, 19) radius 0.5
  circle A468 centre (-1.45, 19) radius 0.5
  circle A469 centre (1.1, 19) radius 0.5
  circle A470 centre (3.65, 19) radius 0.5
  circle A471 centre (6.2, 19) radius 0.5
  circle A472 centre (8.75, 19) radius 0.5
  circle A473 centre (11.3, 19) radius 0.5
  circle A474 centre (13.85, 19) radius 0.5
  circle A475 centre (16.4, 19) radius 0.5
  circle A476 centre (18.95, 19) radius 0.5
  circle A477 centre (21.5, 19) radius 0.5
  circle A478 centre (24.05, 19) radius 0.5
  circle A479 centre (26.6, 19) radius 0.5
  circle A480 centre (29.15, 19) radius 0.5
  circle A481 centre (-29.5, 16.5) radius 0.5
  circle A482 centre (-26.95, 16.5) radius 0.5
  circle A483 centre (-24.4, 16.5) radius 0.5
  circle A484 centre (-21.85, 16.5) radius 0.5
  circle A485 centre (-19.3, 16.5) radius 0.5
  circle A486 centre (-16.75, 16.5) radius 0.5
  circle A487 centre (-14.2, 16.5) radius 0.5
  circle A488 centre (-11.65, 16.5) radius 0.5
  circle A489 centre (-9.1, 16.5) radius 0.5
  circle A490 centre (-6.55, 16.5) radius 0.5
  circle A491 centre (-4, 16.5) radius 0.5
  circle A492 centre (-1.45, 16.5) radius 0.5
  circle A493 centre (1.1, 16.5) radius 0.5
  circle A494 centre (3.65, 16.5) radius 0.5
  circle A495 centre (6.2, 16.5) radius 0.5
  circle A496 centre (8.75, 16.5) radius 0.5
  circle A497 centre (11.3, 16.5) radius 0.5
  circle A498 centre (13.85, 16.5) radius 0.5
  circle A499 centre (16.4, 16.5) radius 0.5
  circle A500 centre (18.95, 16.5) radius 0.5
  circle A501 centre (21.5, 16.5) radius 0.5
  circle A502 centre (24.05, 16.5) radius 0.5
  circle A503 centre (26.6, 16.5) radius 0.5
  circle A504 centre (29.15, 16.5) radius 0.5
  circle A505 centre (-29.5, 14) radius 0.5
  circle A506 centre (-26.95, 14) radius 0.5
  circle A507 centre (-24.4, 14) radius 0.5
  circle A508 centre (-21.85, 14) radius 0.5
  circle A509 centre (-19.3, 14) radius 0.5
  circle A510 centre (-16.75, 14) radius 0.5
  circle A511 centre (-14.2, 14) radius 0.5
  circle A512 centre (-11.65, 14) radius 0.5
  circle A513 centre (-9.1, 14) radius 0.5
  circle A514 centre (-6.55, 14) radius 0.5
  circle A515 centre (-4, 14) radius 0.5
  circle A516 centre (-1.45, 14) radius 0.5
  circle A517 centre (1.1, 14) radius 0.5
  circle A518 centre (3.65, 14) radius 0.5
  circle A519 centre (6.2, 14) radius 0.5
  circle A520 centre (8.75, 14) radius 0.5
  circle A521 centre (11.3, 14) radius 0.5
  circle A522 centre (13.85, 14) radius 0.5
  circle A523 centre (16.4, 14) radius 0.5
  circle A524 centre (18.95, 14) radius 0.5
  circle A525 centre (21.5, 14) radius 0.5
  circle A526 centre (24.05, 14) radius 0.5
  circle A527 centre (26.6, 14) radius 0.5
  circle A528 centre (29.15, 14) radius 0.5
  circle A529 centre (-29.5, 11.5) radius 0.5
  circle A530 centre (-26.95, 11.5) radius 0.5
  circle A531 centre (-24.4, 11.5) radius 0.5
  circle A532 centre (-21.85, 11.5) radius 0.5
  circle A533 centre (-19.3, 11.5) radius 0.5
  circle A534 centre (-16.75, 11.5) radius 0.5
  circle A535 centre (-14.2, 11.5) radius 0.5
  circle A536 centre (-11.65, 11.5) radius 0.5
  circle A537 centre (-9.1, 11.5) radius 0.5
  circle A538 centre (-6.55, 11.5) radius 0.5
  circle A539 centre (-4, 11.5) radius 0.5
  circle A540 centre (-1.45, 11.5) radius 0.5
  circle A541 centre (1.1, 11.5) radius 0.5
  circle A542 centre (3.65, 11.5) radius 0.5
  circle A543 centre (6.2, 11.5) radius 0.5
  circle A544 centre (8.75, 11.5) radius 0.5
  circle A545 centre (11.3, 11.5) radius 0.5
  circle A546 centre (13.85, 11.5) radius 0.5
  circle A547 centre (16.4, 11.5) radius 0.5
  circle A548 centre (18.95, 11.5) radius 0.5
  circle A549 centre (21.5, 11.5) radius 0.5
  circle A550 centre (24.05, 11.5) radius 0.5
  circle A551 centre (26.6, 11.5) radius 0.5
  circle A552 centre (29.15, 11.5) radius 0.5
  circle A553 centre (-29.5, 9) radius 0.5
  circle A554 centre (-26.95, 9) radius 0.5
  circle A555 centre (-24.4, 9) radius 0.5
  circle A556 centre (-21.85, 9) radius 0.5
  circle A557 centre (-19.3, 9) radius 0.5
  circle A558 centre (-16.75, 9) radius 0.5
  circle A559 centre (-14.2, 9) radius 0.5
  circle A560 centre (-11.65, 9) radius 0.5
  circle A561 centre (-9.1, 9) radius 0.5
  circle A562 centre (-6.55, 9) radius 0.5
  circle A563 centre (-4, 9) radius 0.5
  circle A564 centre (-1.45, 9) radius 0.5
  circle A565 centre (1.1, 9) radius 0.5
  circle A566 centre (3.65, 9) radius 0.5
  circle A567 centre (6.2, 9) radius 0.5
  circle A568 centre (8.75, 9) radius 0.5
  circle A569 centre (11.3, 9) radius 0.5
  circle A570 centre (13.85, 9) radius 0.5
  circle A571 centre (16.4, 9) radius 0.5
  circle A572 centre (18.95, 9) radius 0.5
  circle A573 centre (21.5, 9) radius 0.5
  circle A574 centre (24.05, 9) radius 0.5
  circle A575 centre (26.6, 9) radius 0.5
  circle A576 centre (29.15, 9) radius 0.5
  circle A577 centre (-29.5, 6.5) radius 0.5
  circle A578 centre (-26.95, 6.5) radius 0.5
  circle A579 centre (-24.4, 6.5) radius 0.5
  circle A580 centre (-21.85, 6.5) radius 0.5
  circle A581 centre (-19.3, 6.5) radius 0.5
  circle A582 centre (-16.75, 6.5) radius 0.5
  circle A583 centre (-14.2, 6.5) radius 0.5
  circle A584 centre (-11.65, 6.5) radius 0.5
  circle A585 centre (-9.1, 6.5) radius 0.5
  circle A586 centre (-6.55, 6.5) radius 0.5
  circle A587 centre (-4, 6.5) radius 0.5
  circle A588 centre (-1.45, 6.5) radius 0.5
  circle A589 centre (1.1, 6.5) radius 0.5
  circle A590 centre (3.65, 6.5) radius 0.5
  circle A591 centre (6.2, 6.5) radius 0.5
  circle A592 centre (8.75, 6.5) radius 0.5
  circle A593 centre (11.3, 6.5) radius 0.5
  circle A594 centre (13.85, 6.5) radius 0.5
  circle A595 centre (16.4, 6.5) radius 0.5
  circle A596 centre (18.95, 6.5) radius 0.5
  circle A597 centre (21.5, 6.5) radius 0.5
  circle A598 centre (24.05, 6.5) radius 0.5
  circle A599 centre (26.6, 6.5) radius 0.5
  circle A600 centre (29.15, 6.5) radius 0.5
  circle A601 centre (-29.5, 4) radius 0.5
  circle A602 centre (-26.95, 4) radius 0.5
  circle A603 centre (-24.4, 4) radius 0.5
  circle A604 centre (-21.85, 4) radius 0.5
  circle A605 centre (-19.3, 4) radius 0.5
  circle A606 centre (-16.75, 4) radius 0.5
  circle A607 centre (-14.2, 4) radius 0.5
  circle A608 centre (-11.65, 4) radius 0.5
  circle A609 centre (-9.1, 4) radius 0.5
  circle A610 centre (-6.55, 4) radius 0.5
  circle A611 centre (-4, 4) radius 0.5